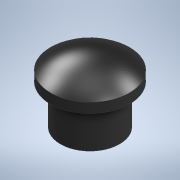
# Autodesk Inventor part: lense
Saved by Autodesk Inventor 2020 (Build 240168000, 168)
## iProperties
Created: 2019-08-05
Part Number: lense
Material: Generic
Document SubType Name: Modeling
Designer: n10208577
Density: 1 g/cm^3
Appearance: Default
Author: n10208577
Autodesk Inventor part; units mm, degrees
ref_plane "YZ Plane" through (0, 0, 0) normal (1, 0, 0) x (0, 1, 0)
ref_plane "XZ Plane" through (0, 0, 0) normal (0, 1, 0) x (-1, 0, 0)
ref_plane "XY Plane" through (0, 0, 0) normal (0, 0, 1) x (1, 0, 0)
sketch "Sketch1" plane through (0, 0, 0) normal (0, 1, 0) x (-1, 0, 0)
  circle A0 centre (0, 0) radius 6
  dimension "d0" = 12
  constraints: 1 centre point, 1 coincident
  measures "d0" diameter of A0
extrude "Extrusion1" add sketch "Sketch1" along normal blind 8
sketch "Sketch2" plane through (0, 8, 0) normal (0, 1, 0) x (1, 0, 0)
  circle A0 centre (0, 0) radius 8
  dimension "d3" = 16
  constraints: 1 centre point, 1 coincident
  measures "d3" diameter of A0
extrude "Extrusion2" add sketch "Sketch2" along normal blind 5
sketch "Sketch3" plane through (0, 0, 0) normal (1, 0, 0) x (0, 1, 0)
  line L0 (13, -8) -> (13, 8) projected
  line L1 (8, -8) -> (8, 8) projected
  line L2 (8, 8) -> (13, 8) projected
  line L3 (8, -8) -> (13, -8) projected
  line L4 (8, 8) -> (10, 8)
  line L5 (10, 8) -> (10, 0)
  line L6 (10, 0) -> (13, 0)
  line L7 (13, -8) -> (13, 8) projected
  line L8 (10, 0) -> (10, -8)
  arc A0 (10, -8) -> (10, 8) centre (0.8333, 0) ccw
  point P0 (0, 0)
  dimension "d6" = 2
  constraints: 8 end point, 3 point on circle, 3 point on line, 1 centre point, 1 midpoint, 1 perpendicular
  measures "d6" distance of L2.start L4.end
revolve "Revolution1" cut sketch "Sketch3" angle 360 about axis through (0, 10, 0) along (0, 1, 0) contours L3 A0 L0 | A0 L2 L0
body "Solid1"
